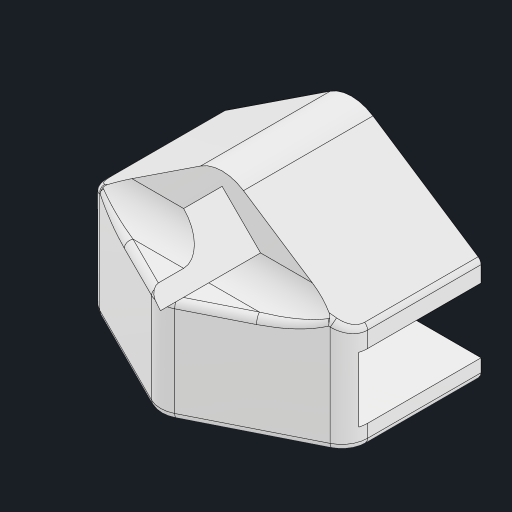
# Autodesk Inventor part: om_TailFrontHolder_FP
Saved by Autodesk Inventor 2023 (Build 270158000, 158)
## iProperties
Created: 2022-06-08
Part Number: om_TailFrontHolder_FP
Material: ABS プラスチック
Document SubType Name: Modeling
Designer: neko2
Density: 1.06 g/cm^3
Appearance: 滑らか - 白
Author: neko2
Autodesk Inventor part; units mm, degrees
ref_plane "YZ Plane" through (0, 0, 0) normal (1, 0, 0) x (0, 1, 0)
ref_plane "XZ Plane" through (0, 0, 0) normal (0, 1, 0) x (-1, 0, 0)
ref_plane "XY Plane" through (0, 0, 0) normal (0, 0, 1) x (1, 0, 0)
sketch "スケッチ1" plane through (0, 0, 0) normal (0, 1, 0) x (-1, 0, 0)
  line L0 (0, 0) -> (0, -14.923)
  line L1 (0, 0) -> (-10, -5)
  line L2 (-10, -5) -> (-10, -15)
  line L3 (-10, -15) -> (0, -15)
  line L4 (0, 0) -> (10, -5)
  line L5 (10, -5) -> (10, -15)
  line L6 (10, -15) -> (0, -15)
  dimension "d0" = 20
  dimension "d1" = 5
  dimension "d2" = 15
  constraints: 14 end point, 2 symmetric about line, 2 vertical, 1 perpendicular, 1 point on line
  measures "d0" diameter of L2 L0
  measures "d1" vertical distance of L0.start L1.end
  measures "d2" distance from line of L0.start L3
extrude "押し出し1" add sketch "スケッチ1" along normal blind 1.5
sketch "スケッチ2" plane through (0, 1.5, 0) normal (0, 1, 0) x (1, 0, 0)
  line L0 (0, 0) -> (10, 5) projected
  line L1 (0, 0) -> (0, 15)
  line L2 (10, 15) -> (-10, 15) projected
  line L3 (0, 3) -> (150, 43)
  line L4 (10, 15) -> (-10, 15) projected
  line L5 (-10, 15) -> (-10, 5) projected
  line L6 (-10, 5) -> (0, 0) projected
  line L7 (0, 0) -> (10, 5) projected
  line L8 (10, 5) -> (10, 15) projected
  line L9 (0, 3) -> (-150, 43)
  point P0 (10, 5.6667)
  point P1 (-10, 5.6667)
  dimension "d5" = 300
  dimension "d6" = 40
  dimension "d7" = 3
  constraints: 6 end point, 1 midpoint, 1 point on line, 1 symmetric about line
  measures "d5" diameter of L3.end L1
  measures "d6" vertical distance of L3.end L3.start
  measures "d7" distance of L0.start L3.start
extrude "押し出し2" add sketch "スケッチ2" along normal blind 5 contours L1 L3 L8 L0 | L6 L5 L9 L1
sketch "スケッチ3" plane through (0, 6.5, 0) normal (0, 1, 0) x (1, 0, 0)
  line L0 (0, 0) -> (10, 5) projected
  line L1 (10, 5) -> (10, 5.6667) projected
  line L2 (10, 5.6667) -> (0, 3) projected
  line L3 (0, 3) -> (-10, 5.6667) projected
  line L4 (-10, 5.6667) -> (-10, 5) projected
  line L5 (-10, 5) -> (0, 0) projected
  line L6 (0, 3) -> (10, 5.6667) projected
  line L7 (10, 5.6667) -> (10, 15) projected
  line L8 (10, 15) -> (-10, 15) projected
  line L9 (-10, 15) -> (-10, 5.6667) projected
  line L10 (-10, 5.6667) -> (0, 3) projected
  line L11 (-10, 15) -> (-10, 5.6667) projected
  line L12 (-10, 15) -> (10, 15)
  line L13 (10, 5) -> (10, 15) projected
  point P0 (10, 15)
  dimension "d10" = 15
  constraints: 2 end point, 2 point on line, 1 perpendicular
  measures "d10" distance from line of L12 point (0, 0)
extrude "押し出し3" add sketch "スケッチ3" along normal blind 1.5
sketch "スケッチ4" plane through (10, 6.5, -15) normal (0, 0, -1) x (-1, 0, 0)
  circle A0 centre (10, 4.5) radius 3
  line L0 (0, 1.5) -> (20, 1.5) projected
  line L1 (8.3486, 7.0046) -> (0, 1.5)
  line L2 (11.6514, 7.0046) -> (20, 1.5)
  line L3 (0, 0) -> (20, 0) projected
  line L4 (20, 0) -> (20, 1.5) projected
  line L5 (0, 1.5) -> (20, 1.5) projected
  line L6 (0, 0) -> (0, 1.5) projected
  point P0 (10, -6.5)
  point P1 (10, 1.5)
  point P2 (10, 0)
  dimension "d13" = 6
  dimension "d15" = 10
  dimension "d17" = 10
  constraints: 4 end point, 3 point on circle, 3 tangent, 2 midpoint, 2 point on line, 1 centre point
  measures "d13" diameter of A0
  measures "d15" distance of A0.start L1.end
  measures "d17" distance of L2.end A0.start
extrude "押し出し4" add sketch "スケッチ4" against normal blind 10 contours A0 | A0 L2 L0 | L0 L1 A0
fillet "フィレット2" radius 2 1 edges at (0, 8, -5)
fillet "フィレット3" radius 2 3 edges at (-10, 4, -5) (0, 4, 0) (10, 4, -5)
fillet "フィレット4" radius 0.5 12 edges at (0, 8, -0.2361) (3.4472, 8, -1.7236) (10, 8, -10.618) (-10, 8, -10.618) (-3.4472, 8, -1.7236) (0, 0, -0.2361) (4.8944, 0, -2.4472) (9.7013, 0, -5.1846) (10, 0, -10.618) (-9.7013, 0, -5.1846) (-10, 0, -10.618) (-4.8944, 0, -2.4472)
sketch "スケッチ5" plane through (10, 6.5, -15) normal (0, 0, -1) x (-1, 0, 0)
  arc A0 (0.2248, 1.6482) -> (0, 1.2308) centre (0.5, 1.2308) ccw projected
  line L0 (0, 0) -> (0, 1.2308) projected
  line L1 (0, 0) -> (20, 0) projected
  line L2 (20, 0) -> (20, 1.2308) projected
  arc A1 (20, 1.2308) -> (19.7752, 1.6482) centre (19.5, 1.2308) ccw projected
  line L3 (19.7752, 1.6482) -> (11.6514, 7.0046) projected
  arc A2 (11.6514, 7.0046) -> (8.3486, 7.0046) centre (10, 4.5) ccw projected
  line L4 (8.3486, 7.0046) -> (0.2248, 1.6482) projected
  line L5 (10, -5) -> (10, 0) projected
  line L6 (7.0302, 3.5) -> (10, 6.4698)
  line L7 (10, 6.4698) -> (12.9698, 3.5)
  line L8 (12.9698, 3.5) -> (10, 0.5302)
  line L9 (10, 0.5302) -> (7.0302, 3.5)
  line L10 (0, 0) -> (20, 0) projected
  point P0 (10, -6.5)
  point P1 (10, 0)
  point P2 (10, 3.5)
  point P3 (10, 0)
  dimension "d29" = 4.2
  dimension "d31" = 3.5
  constraints: 8 end point, 3 vertical alignment, 2 midpoint, 2 parallel, 2 perpendicular, 1 horizontal alignment
  measures "d29" distance of L6.start L6.end
  measures "d31" distance of point (10, 3.5) point (10, 0)
extrude "押し出し5" cut sketch "スケッチ5" against normal through all contours L6 L7 L8 L9
ref_plane "作業平面1" through (-2.9698, 10, -15) normal (0, 1, 0) x (0, 0, 1)
